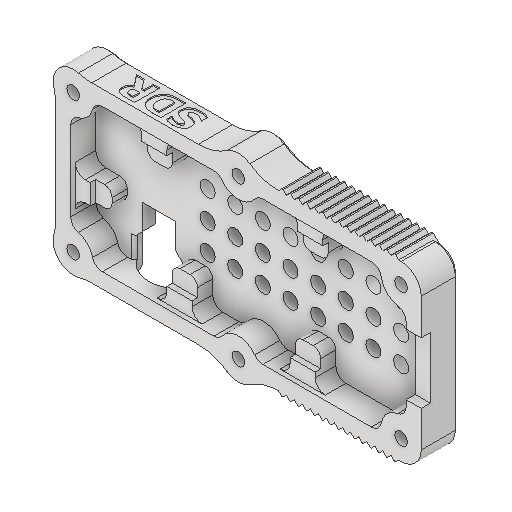
# Autodesk Inventor part: 3DP_PLA_Case_bottom_half
Saved by Autodesk Inventor 2025 (Build 290162010, 162A)
## iProperties
Created: 2018-09-08
Part Number: 3DP_PLA_Case_bottom_half
Material: ABS Plastic
Document SubType Name: Modeling
Designer: Andrzej
Density: 1.06 g/cm^3
Appearance: Smooth - White
Author: Andrzej
Autodesk Inventor part; units mm, degrees
ref_plane "YZ Plane" through (0, 0, 0) normal (1, 0, 0) x (0, 1, 0)
ref_plane "XZ Plane" through (0, 0, 0) normal (0, 1, 0) x (-1, 0, 0)
ref_plane "XY Plane" through (0, 0, 0) normal (0, 0, 1) x (1, 0, 0)
sketch "Sketch1" plane through (0, 0, 0) normal (0, 0, 1) x (1, 0, 0)
  line L0 (-16.557, 11) -> (35.343, 11)
  line L1 (35.343, -11) -> (-16.557, -11)
  line L2 (-20.157, -7.4) -> (-20.157, 7.4)
  line L3 (38.843, 7) -> (46.2445, 7)
  line L4 (46.2445, 7) -> (46.2445, -7)
  line L5 (46.2445, -7) -> (38.843, -7)
  arc A0 (-20.157, -7.4) -> (-16.557, -11) centre (-16.557, -7.4) ccw
  arc A1 (-16.557, 11) -> (-20.157, 7.4) centre (-16.557, 7.4) ccw
  arc A2 (37.843, 8.5) -> (35.343, 11) centre (35.343, 8.5) ccw
  arc A3 (35.343, -11) -> (37.843, -8.5) centre (35.343, -8.5) ccw
  line L6 (37.843, 8.5) -> (37.843, 8)
  line L7 (37.843, -8) -> (37.843, -8.5)
  arc A4 (37.843, 8) -> (38.843, 7) centre (38.843, 8) ccw
  arc A5 (38.843, -7) -> (37.843, -8) centre (38.843, -8) ccw
  circle A6 centre (-17.157, -8) radius 1.05
  circle A7 centre (-15.157, 9.4) radius 1.05
  line L8 (-5.157, -11) -> (-0.157, -11)
  line L9 (-0.157, -11) -> (-0.157, -8)
  line L10 (-0.157, -8) -> (-5.157, -8)
  line L11 (-5.157, -8) -> (-5.157, -11)
  line L12 (19.343, -11) -> (24.343, -11)
  line L13 (24.343, -11) -> (24.343, -8)
  line L14 (24.343, -8) -> (19.343, -8)
  line L15 (19.343, -8) -> (19.343, -11)
  line L16 (-10.157, 11) -> (-5.157, 11)
  line L17 (-5.157, 11) -> (-5.157, 8)
  line L18 (-5.157, 8) -> (-10.157, 8)
  line L19 (-10.157, 8) -> (-10.157, 11)
  line L20 (20.843, 11) -> (25.843, 11)
  line L21 (25.843, 11) -> (25.843, 8)
  line L22 (25.843, 8) -> (20.843, 8)
  line L23 (20.843, 8) -> (20.843, 11)
  line L24 (-10.157, 11) -> (-5.157, 11)
  line L25 (-5.157, 11) -> (-5.157, 11.25)
  line L26 (-5.157, 11.25) -> (-10.157, 11.25)
  line L27 (-10.157, 11.25) -> (-10.157, 11)
  line L28 (20.843, 11) -> (25.843, 11)
  line L29 (25.843, 11) -> (25.843, 11.25)
  line L30 (25.843, 11.25) -> (20.843, 11.25)
  line L31 (20.843, 11.25) -> (20.843, 11)
  line L32 (-5.157, -11) -> (-0.157, -11)
  line L33 (-0.157, -11) -> (-0.157, -11.25)
  line L34 (-0.157, -11.25) -> (-5.157, -11.25)
  line L35 (-5.157, -11.25) -> (-5.157, -11)
  line L36 (19.343, -11) -> (24.343, -11)
  line L37 (24.343, -11) -> (24.343, -11.25)
  line L38 (24.343, -11.25) -> (19.343, -11.25)
  line L39 (19.343, -11.25) -> (19.343, -11)
  line L40 (-5.157, -11.25) -> (-0.157, -11.25)
  line L41 (-0.157, -11.25) -> (-0.157, -14.25)
  line L42 (-0.157, -14.25) -> (-5.157, -14.25)
  line L43 (-5.157, -14.25) -> (-5.157, -11.25)
  line L44 (19.343, -11.25) -> (24.343, -11.25)
  line L45 (24.343, -11.25) -> (24.343, -14.25)
  line L46 (24.343, -14.25) -> (19.343, -14.25)
  line L47 (19.343, -14.25) -> (19.343, -11.25)
  line L48 (-10.157, 11.25) -> (-5.157, 11.25)
  line L49 (-5.157, 11.25) -> (-5.157, 14.25)
  line L50 (-5.157, 14.25) -> (-10.157, 14.25)
  line L51 (-10.157, 14.25) -> (-10.157, 11.25)
  line L52 (20.843, 11.25) -> (25.843, 11.25)
  line L53 (25.843, 11.25) -> (25.843, 14.25)
  line L54 (25.843, 14.25) -> (20.843, 14.25)
  line L55 (20.843, 14.25) -> (20.843, 11.25)
  line L56 (-20.157, -5) -> (-17.157, -5)
  line L57 (-17.157, -5) -> (-17.157, -1)
  line L58 (-17.157, -1) -> (-20.157, -1)
  line L59 (-20.157, -1) -> (-20.157, -5)
  line L60 (-20.157, -5) -> (-20.407, -5)
  line L61 (-20.407, -5) -> (-20.407, -1)
  line L62 (-20.407, -1) -> (-20.157, -1)
  line L63 (-20.157, -1) -> (-20.157, -5)
  line L64 (-20.407, -1) -> (-23.407, -1)
  line L65 (-23.407, -1) -> (-23.407, -5)
  line L66 (-23.407, -5) -> (-20.407, -5)
  line L67 (-20.407, -5) -> (-20.407, -1)
  point P0 (0, 0)
  point P1 (0, 0)
  dimension "d0" = 14
  dimension "d1" = 4
  dimension "d2" = 3.6
  dimension "d3" = 2.5
  dimension "d4" = 1
  dimension "d5" = 2.1
  dimension "d6" = 3
  dimension "d7" = 3
  dimension "d8" = 2.1
  dimension "d9" = 5
  dimension "d10" = 1.6
  dimension "d12" = 5
  dimension "d13" = 3
  dimension "d14" = 5
  dimension "d15" = 3
  dimension "d16" = 5
  dimension "d17" = 3
  dimension "d18" = 5
  dimension "d19" = 3
  dimension "d20" = 15
  dimension "d21" = 10
  dimension "d22" = 5
  dimension "d23" = 0.25
  dimension "d24" = 5
  dimension "d25" = 0.25
  dimension "d27" = 5
  dimension "d28" = 0.25
  dimension "d29" = 5
  dimension "d30" = 0.25
  dimension "d31" = 3
  dimension "d32" = 5
  dimension "d33" = 3
  dimension "d34" = 5
  dimension "d35" = 3
  dimension "d36" = 5
  dimension "d37" = 3
  dimension "d42" = 22
  dimension "d43" = 3
  dimension "d44" = 4
  dimension "d45" = 0.25
  dimension "d46" = 3
  dimension "d47" = 6
  dimension "d69" = 58
  dimension "d70" = 12
  dimension "d71" = 5
  dimension "d72" = 13.5
  dimension "d148" = 11
  constraints: 136 end point, 33 parallel, 20 perpendicular, 17 horizontal, 14 tangent, 12 point on circle, 8 centre point, 7 point on line, 3 equal radius
  measures "d0" distance of L3.end L4.end
  measures "d1" distance between parallel lines of L0 L3
  measures "d2" radius of A0
  measures "d3" radius of A2
  measures "d4" radius of A4
  measures "d5" diameter of A6
  measures "d6" distance from line of L1 A6.centre
  measures "d7" distance from line of L2 A6.centre
  measures "d8" diameter of A7
  measures "d9" distance from line of L2 A7.centre
  measures "d10" distance from line of L0 A7.centre
  measures "d12" distance of L10.end L9.end
  measures "d13" distance of L9.end L8.end
  measures "d14" distance of L14.end L13.end
  measures "d15" distance of L13.end L12.end
  measures "d16" distance of L17.end L18.end
  measures "d17" distance of L16.end L17.end
  measures "d18" distance of L21.end L22.end
  measures "d19" distance of L20.end L21.end
  measures "d20" distance between parallel lines of L2 L11
  measures "d21" distance between parallel lines of L2 L19
  measures "d22" distance of L26.end L25.end
  measures "d23" distance of L25.end L24.end
  measures "d24" distance of L30.end L29.end
  measures "d25" distance of L29.end L28.end
  measures "d27" distance of L33.end L34.end
  measures "d28" distance of L32.end L33.end
  measures "d29" distance of L37.end L38.end
  measures "d30" distance of L36.end L37.end
  measures "d31" distance of L40.end L41.end
  measures "d32" distance of L45.end L46.end
  measures "d33" distance of L44.end L45.end
  measures "d34" distance of L50.end L49.end
  measures "d35" distance of L49.end L48.end
  measures "d36" distance of L54.end L53.end
  measures "d37" distance of L53.end L52.end
  measures "d42" distance between parallel lines of L1 L0
  measures "d43" distance of L58.end L57.end
  measures "d44" distance of L57.end L56.end
  measures "d45" distance of L61.end L62.end
  measures "d46" distance of L66.end L65.end
  measures "d47" distance between parallel lines of L1 L56
  measures "d69" distance between parallel lines of L2 L6
  measures "d70" distance between parallel lines of L6 L21
  measures "d71" distance of L41.end L42.end
  measures "d72" distance between parallel lines of L7 L13
  measures "d148" distance from line of point (0, 0) L0
extrude "Extrusion1" add sketch "Sketch1" against normal blind 3 contours L27 L26 L25 L0 | L0 L17 L18 L19 | L51 L50 L49 L26 | L58 L57 L56 L2 | L2 L60 L61 L62 | L31 L30 L29 L0 | L0 L21 L22 L23 | L61 L66 L65 L64 | L55 L54 L53 L30 | L11 L10 L9 L1 | L1 L33 L34 L35 | L34 L41 L42 L43 | L15 L14 L13 L1 | L1 L37 L38 L39 | L38 L45 L46 L47
extrude "Extrusion2" add sketch "Sketch1" along normal blind 1.1 contours L51 L50 L49 L26 | L61 L66 L65 L64 | L55 L54 L53 L30 | L34 L41 L42 L43 | L38 L45 L46 L47
sketch "Sketch2" plane through (0, 0, -3) normal (0, 0, -1) x (-1, 0, 0)
  line L0 (17.157, -5) -> (23.407, -5) projected
  line L1 (23.407, -5) -> (23.407, -1) projected
  line L2 (23.407, -1) -> (17.157, -1) projected
  line L3 (17.157, -1) -> (17.157, -5) projected
  line L4 (5.157, -14.25) -> (5.157, -8) projected
  line L5 (5.157, -8) -> (0.157, -8) projected
  line L6 (0.157, -8) -> (0.157, -14.25) projected
  line L7 (0.157, -14.25) -> (5.157, -14.25) projected
  line L8 (-19.343, -14.25) -> (-19.343, -8) projected
  line L9 (-19.343, -8) -> (-24.343, -8) projected
  line L10 (-24.343, -8) -> (-24.343, -14.25) projected
  line L11 (-24.343, -14.25) -> (-19.343, -14.25) projected
  line L12 (-20.843, 8) -> (-20.843, 14.25) projected
  line L13 (-20.843, 14.25) -> (-25.843, 14.25) projected
  line L14 (-25.843, 14.25) -> (-25.843, 8) projected
  line L15 (-25.843, 8) -> (-20.843, 8) projected
  line L16 (10.157, 8) -> (10.157, 14.25) projected
  line L17 (10.157, 14.25) -> (5.157, 14.25) projected
  line L18 (5.157, 14.25) -> (5.157, 8) projected
  line L19 (5.157, 8) -> (10.157, 8) projected
  line L20 (23.407, 14.25) -> (-46.343, 14.25)
  line L21 (-46.343, 14.25) -> (-46.343, -14.25)
  line L22 (-46.343, -14.25) -> (23.407, -14.25)
  line L23 (23.407, -14.25) -> (23.407, 14.25)
  line L24 (23.407, -5) -> (23.407, -1) projected
  line L25 (0.157, -14.25) -> (5.157, -14.25) projected
  line L26 (-46.343, -14.25) -> (-46.343, -17.25)
  line L27 (-46.343, -17.25) -> (26.407, -17.25)
  line L28 (26.407, -17.25) -> (26.407, 17.25)
  line L29 (26.407, 17.25) -> (-46.343, 17.25)
  line L30 (-46.343, 17.25) -> (-46.343, 14.25)
  dimension "d49" = 28.5
  dimension "d50" = 47.75
  dimension "d51" = 28.5
  dimension "d52" = 69.75
  dimension "d53" = 3
  dimension "d54" = 3
  dimension "d55" = 3
  constraints: 18 end point, 4 perpendicular, 3 collinear, 2 parallel, 1 horizontal, 1 point on line, 1 vertical
  measures "d49" distance between parallel lines of L17 L7
  measures "d50" distance between parallel lines of L10 L1
  measures "d51" distance of L20.end L21.end
  measures "d52" distance of L21.end L22.end
  measures "d53" distance between parallel lines of L27 L22
  measures "d54" distance between parallel lines of L20 L29
  measures "d55" distance between parallel lines of L28 L23
extrude "Extrusion3" add sketch "Sketch2" along normal blind 2.5
sketch "Sketch3" plane through (0, 0, -3) normal (0, 0, 1) x (1, 0, 0)
  line L0 (46.343, 17.25) -> (46.343, -17.25) projected
  line L1 (-26.407, 17.25) -> (46.343, 17.25) projected
  line L2 (-26.407, -17.25) -> (-26.407, 17.25) projected
  line L3 (46.343, -17.25) -> (-26.407, -17.25) projected
  line L4 (24.343, -14.25) -> (19.343, -14.25) projected
  line L5 (19.343, -14.25) -> (19.343, -8) projected
  line L6 (19.343, -8) -> (24.343, -8) projected
  line L7 (24.343, -8) -> (24.343, -14.25) projected
  line L8 (-10.157, 14.25) -> (-5.157, 14.25) projected
  line L9 (-5.157, 14.25) -> (-5.157, 8) projected
  line L10 (-5.157, 8) -> (-10.157, 8) projected
  line L11 (-10.157, 8) -> (-10.157, 14.25) projected
  line L12 (-23.407, -5) -> (-23.407, -1) projected
  line L13 (-23.407, -1) -> (-17.157, -1) projected
  line L14 (-17.157, -1) -> (-17.157, -5) projected
  line L15 (-17.157, -5) -> (-23.407, -5) projected
  line L16 (20.843, 14.25) -> (25.843, 14.25) projected
  line L17 (25.843, 14.25) -> (25.843, 8) projected
  line L18 (25.843, 8) -> (20.843, 8) projected
  line L19 (20.843, 8) -> (20.843, 14.25) projected
  line L20 (-0.157, -14.25) -> (-5.157, -14.25) projected
  line L21 (-5.157, -14.25) -> (-5.157, -8) projected
  line L22 (-5.157, -8) -> (-0.157, -8) projected
  line L23 (-0.157, -8) -> (-0.157, -14.25) projected
  line L24 (43.343, 14.25) -> (43.343, -14.25)
  line L25 (43.343, -14.25) -> (-23.407, -14.25)
  line L26 (-23.407, -14.25) -> (-23.407, 14.25)
  line L27 (-23.407, 14.25) -> (43.343, 14.25)
  dimension "d58" = 3
  constraints: 8 end point, 3 other
  measures "d58" distance between parallel lines of L1 L27
extrude "Extrusion4" add sketch "Sketch3" along normal blind 5
fillet "Fillet1" radius 6 4 edges at (-23.407, 14.25, -0.5) (-26.407, 17.25, -1.75) (-23.407, -14.25, -0.5) (-26.407, -17.25, -1.75)
fillet "Fillet1" radius 4 4 edges at (43.343, 14.25, -0.5) (46.343, 17.25, -1.75) (46.343, -17.25, -1.75) (43.343, -14.25, -0.5)
sketch "Sketch5" plane through (0, 0, 2) normal (0, 0, 1) x (1, 0, 0)
  line L0 (39.343, -14.25) -> (-17.407, -14.25) projected
  arc A0 (-23.407, -8.25) -> (-17.407, -14.25) centre (-17.407, -8.25) ccw projected
  line L1 (-23.407, -8.25) -> (-23.407, 8.25) projected
  arc A1 (-17.407, 14.25) -> (-23.407, 8.25) centre (-17.407, 8.25) ccw projected
  line L2 (-17.407, 14.25) -> (39.343, 14.25) projected
  arc A2 (43.343, 10.25) -> (39.343, 14.25) centre (39.343, 10.25) ccw projected
  line L3 (43.343, 10.25) -> (43.343, -10.25) projected
  arc A3 (39.343, -14.25) -> (43.343, -10.25) centre (39.343, -10.25) ccw projected
  arc A4 (42.343, -17.25) -> (46.343, -13.25) centre (42.343, -13.25) ccw projected
  line L4 (46.343, -13.25) -> (46.343, 13.25) projected
  arc A5 (46.343, 13.25) -> (42.343, 17.25) centre (42.343, 13.25) ccw projected
  line L5 (42.343, 17.25) -> (-20.407, 17.25) projected
  arc A6 (-20.407, 17.25) -> (-26.407, 11.25) centre (-20.407, 11.25) ccw projected
  line L6 (-26.407, 11.25) -> (-26.407, -11.25) projected
  arc A7 (-26.407, -11.25) -> (-20.407, -17.25) centre (-20.407, -11.25) ccw projected
  line L7 (-20.407, -17.25) -> (42.343, -17.25) projected
  circle A8 centre (42.343, -13.25) radius 4
  circle A9 centre (9.968, -15.75) radius 4
  circle A10 centre (-22.907, -13.75) radius 4
  circle A11 centre (42.343, 13.25) radius 4
  circle A12 centre (9.968, 15.75) radius 4
  circle A13 centre (-22.907, 13.75) radius 4
  point P0 (0, 0)
  dimension "d73" = 8
  dimension "d74" = 8
  dimension "d75" = 8
  dimension "d76" = 36.375
  dimension "d77" = 72.75
  dimension "d78" = 1.5
  dimension "d79" = 8
  dimension "d80" = 8
  dimension "d81" = 8
  dimension "d82" = 3.5
  dimension "d83" = 3.5
  dimension "d84" = 3.5
  dimension "d85" = 1.5
  constraints: 6 centre point, 2 coincident, 2 vertical alignment
  measures "d73" diameter of A8
  measures "d74" diameter of A9
  measures "d75" diameter of A10
  measures "d76" distance from line of L4 A9.centre
  measures "d77" distance between parallel lines of L4 L6
  measures "d78" distance from line of L7 A9.centre
  measures "d79" diameter of A11
  measures "d80" diameter of A12
  measures "d81" diameter of A13
  measures "d82" distance from line of A10.centre L7
  measures "d83" distance from line of A10.centre L6
  measures "d84" distance from line of L5 A13.centre
  measures "d85" distance from line of L5 A12.centre
extrude "Extrusion5" add sketch "Sketch5" against normal up to surface (7.5 mm away) contours A3 L3 A8 A4 L0 | L0 A8 L3 A3 | A9 L7 L0 | L0 A9 | A11 L2 A2 L3 | L3 A2 L2 A11 A5 | A9 L7 | A10 A7 A0 | A0 A10 | A12 L2 | L2 A12 L5 | A10 A7 | L5 A12 | A13 A1 | A1 A13 A6 | A6 A13
hole "Hole1" at (-22.907, -13.75, 2) at (9.968, -15.75, 2) at (42.343, -13.25, 2) at (9.968, 15.75, 2) at (42.343, 13.25, 2) at (-22.907, 13.75, 2) direction (0, 0, -1) diameter 2.5 end through all both
sketch "Sketch6" plane through (46.343, -13.25, -5.5) normal (1, 0, 0) x (0, 0, -1)
  line L0 (0, 0) -> (-7.5, 0) projected
  line L1 (0, 26.5) -> (0, 0) projected
  line L2 (-7.5, 26.5) -> (0, 26.5) projected
  line L3 (-7.5, 0) -> (-7.5, 26.5) projected
  line L4 (-7.5, 22.627) -> (-7.5, 3.873) projected
  line L5 (-7.5, 7.175) -> (-5.7, 7.175)
  line L6 (-5.7, 7.175) -> (-5.7, 19.325)
  line L7 (-5.7, 19.325) -> (-7.5, 19.325)
  line L8 (-7.5, 7.175) -> (-7.5, 19.325)
  point P0 (-5.5, 13.25)
  dimension "d95" = 1.8
  dimension "d96" = 12.15
  dimension "d97" = 26.5
  dimension "d98" = 7.175
  constraints: 8 end point, 2 perpendicular, 2 point on line, 1 collinear, 1 horizontal
  measures "d95" distance of L5.start L5.end
  measures "d96" distance of L5.end L6.end
  measures "d97" distance between parallel lines of L2 L0
  measures "d98" distance between parallel lines of L0 L5
extrude "Extrusion6" cut sketch "Sketch6" against normal blind 6 contours L3 L7 L6 L5
fillet "Fillet2" radius 2 10 edges at (-10.157, 14.25, -0.95) (-5.157, 14.25, -0.95) (20.843, 14.25, -0.95) (25.843, 14.25, -0.95) (19.343, -14.25, -0.95) (24.343, -14.25, -0.95) (-0.157, -14.25, -0.95) (-5.157, -14.25, -0.95) (-23.407, -1, -0.95) (-23.407, -5, -0.95)
fillet "Fillet2" radius 1.5 10 edges at (-10.157, 8, -1.5) (-5.157, 8, -1.5) (20.843, 8, -1.5) (25.843, 8, -1.5) (-17.157, -5, -1.5) (-17.157, -1, -1.5) (-5.157, -8, -1.5) (-0.157, -8, -1.5) (19.343, -8, -1.5) (24.343, -8, -1.5)
sketch "Sketch7" plane through (-20.407, -17.25, -5.5) normal (0, -1, 0) x (1, 0, 0)
  circle A0 centre (9.5728, -1.45) radius 6
  line L0 (26.6669, 0) -> (0, 0) projected
  line L1 (-5.9772, 0) -> (-5.9772, 7.5) projected
  point P0 (20.407, 5.5)
  dimension "d103" = 12
  dimension "d104" = 1.45
  dimension "d105" = 15.55
  constraints: 1 centre point
  measures "d103" diameter of A0
  measures "d104" distance from line of L0 A0.centre
  measures "d105" distance from line of L1 A0.centre
extrude "Extrusion7" cut sketch "Sketch7" against normal blind 7.45
sketch "Sketch8" plane through (0, 0, -5.5) normal (0, 0, -1) x (-1, 0, 0)
  line L0 (5.012, -17.25) -> (5.012, -9.8) projected
  line L1 (5.012, -9.8) -> (16.6563, -9.8) projected
  line L2 (16.6563, -9.8) -> (16.6563, -17.25) projected
  line L3 (16.6563, -17.25) -> (20.407, -17.25) projected
  arc A0 (20.407, -17.25) -> (20.9298, -17.2272) centre (20.407, -11.25) ccw projected
  arc A1 (20.9298, -17.2272) -> (26.3842, -11.7728) centre (22.907, -13.75) ccw projected
  arc A2 (26.3842, -11.7728) -> (26.407, -11.25) centre (20.407, -11.25) ccw projected
  line L4 (26.407, -11.25) -> (26.407, 11.25) projected
  arc A3 (26.407, 11.25) -> (26.3842, 11.7728) centre (20.407, 11.25) ccw projected
  arc A4 (26.3842, 11.7728) -> (20.9298, 17.2272) centre (22.907, 13.75) ccw projected
  arc A5 (20.9298, 17.2272) -> (20.407, 17.25) centre (20.407, 11.25) ccw projected
  line L5 (20.407, 17.25) -> (-6.2599, 17.25) projected
  arc A6 (-6.2599, 17.25) -> (-13.6761, 17.25) centre (-9.968, 15.75) ccw projected
  line L6 (-13.6761, 17.25) -> (-42.343, 17.25) projected
  arc A7 (-42.343, 17.25) -> (-46.343, 13.25) centre (-42.343, 13.25) ccw projected
  line L7 (-46.343, 13.25) -> (-46.343, -13.25) projected
  arc A8 (-46.343, -13.25) -> (-42.343, -17.25) centre (-42.343, -13.25) ccw projected
  line L8 (-42.343, -17.25) -> (-13.6761, -17.25) projected
  arc A9 (-13.6761, -17.25) -> (-6.2599, -17.25) centre (-9.968, -15.75) ccw projected
  line L9 (-6.2599, -17.25) -> (5.012, -17.25) projected
  circle A10 centre (22.907, 13.75) radius 1.25 projected
  circle A11 centre (-9.968, 15.75) radius 1.25 projected
  circle A12 centre (-9.968, -15.75) radius 1.25 projected
  circle A13 centre (22.907, -13.75) radius 1.25 projected
  circle A14 centre (-42.343, -13.25) radius 1.25 projected
  circle A15 centre (-42.343, 13.25) radius 1.25 projected
  line L10 (14.0842, -9.8) -> (7.5842, -9.8)
  line L11 (7.5842, -9.8) -> (7.5842, -3.3)
  line L12 (7.5842, -3.3) -> (14.0842, -3.3)
  line L13 (14.0842, -3.3) -> (14.0842, -9.8)
  point P0 (0, 0)
  dimension "d108" = 6.5
  dimension "d109" = 6.5
  dimension "d110" = 11.6443
  dimension "d111" = 2.5722
  constraints: 8 end point, 2 parallel, 1 horizontal, 1 perpendicular, 1 point on line
  measures "d108" distance of L11.end L12.end
  measures "d109" distance of L10.end L11.end
  measures "d110" distance between parallel lines of L0 L2
  measures "d111" distance between parallel lines of L2 L13
extrude "Extrusion8" cut sketch "Sketch8" against normal blind 8 contours L11 L12 L13 L1
fillet "Fillet3" radius 0.5 2 edges at (-15.3505, -12.025, -3) (-6.3178, -11.9327, -3)
chamfer "Chamfer1" distance 1.5 angle 45 2 edges at (-7.5842, -9.8, -4.25) (-14.0842, -9.8, -4.25)
fillet "Fillet4" radius 10 8 edges at (-26.3842, -11.7728, -1.75) (-26.3842, 11.7728, -1.75) (-20.9298, -17.2272, -1.75) (6.2599, -17.25, -1.75) (13.6761, -17.25, -1.75) (13.6761, 17.25, -1.75) (6.2599, 17.25, -1.75) (-20.9298, 17.2272, -1.75)
sketch "Sketch9" plane through (0, 0, -3) normal (0, 0, 1) x (1, 0, 0)
  line L0 (-14.0842, -8.3) -> (-15.5842, -9.8) projected
  line L1 (-14.0842, -8.3) -> (-14.0842, -3.3) projected
  line L2 (-14.0842, -3.3) -> (-7.5842, -3.3) projected
  line L3 (-7.5842, -3.3) -> (-7.5842, -8.3) projected
  line L4 (-6.0842, -9.8) -> (-7.5842, -8.3) projected
  line L5 (-6.0842, -9.8) -> (-5.3253, -9.8) projected
  line L6 (-5.3253, -13.0531) -> (-5.3253, -9.8) projected
  arc A0 (-5.3253, -13.0531) -> (-5.157, -12.25) centre (-7.157, -12.25) ccw projected
  line L7 (-5.157, -12.25) -> (-5.157, -9.5) projected
  arc A1 (-3.657, -8) -> (-5.157, -9.5) centre (-3.657, -9.5) ccw projected
  line L8 (-3.657, -8) -> (-1.657, -8) projected
  arc A2 (-0.157, -9.5) -> (-1.657, -8) centre (-1.657, -9.5) ccw projected
  line L9 (-0.157, -9.5) -> (-0.157, -12.25) projected
  arc A3 (-0.157, -12.25) -> (1.843, -14.25) centre (1.843, -12.25) ccw projected
  line L10 (1.843, -14.25) -> (6.2599, -14.25) projected
  arc A4 (13.6761, -14.25) -> (6.2599, -14.25) centre (9.968, -15.75) ccw projected
  line L11 (13.6761, -14.25) -> (17.343, -14.25) projected
  arc A5 (17.343, -14.25) -> (19.343, -12.25) centre (17.343, -12.25) ccw projected
  line L12 (19.343, -12.25) -> (19.343, -9.5) projected
  arc A6 (20.843, -8) -> (19.343, -9.5) centre (20.843, -9.5) ccw projected
  line L13 (20.843, -8) -> (22.843, -8) projected
  arc A7 (24.343, -9.5) -> (22.843, -8) centre (22.843, -9.5) ccw projected
  line L14 (24.343, -9.5) -> (24.343, -12.25) projected
  arc A8 (24.343, -12.25) -> (26.343, -14.25) centre (26.343, -12.25) ccw projected
  line L15 (26.343, -14.25) -> (38.47, -14.25) projected
  arc A9 (43.343, -9.377) -> (38.47, -14.25) centre (42.343, -13.25) ccw projected
  line L16 (43.343, -9.377) -> (43.343, 9.377) projected
  arc A10 (38.47, 14.25) -> (43.343, 9.377) centre (42.343, 13.25) ccw projected
  line L17 (38.47, 14.25) -> (27.843, 14.25) projected
  arc A11 (27.843, 14.25) -> (25.843, 12.25) centre (27.843, 12.25) ccw projected
  line L18 (25.843, 12.25) -> (25.843, 9.5) projected
  arc A12 (24.343, 8) -> (25.843, 9.5) centre (24.343, 9.5) ccw projected
  line L19 (24.343, 8) -> (22.343, 8) projected
  arc A13 (20.843, 9.5) -> (22.343, 8) centre (22.343, 9.5) ccw projected
  line L20 (20.843, 9.5) -> (20.843, 12.25) projected
  arc A14 (20.843, 12.25) -> (18.843, 14.25) centre (18.843, 12.25) ccw projected
  line L21 (18.843, 14.25) -> (13.6761, 14.25) projected
  arc A15 (6.2599, 14.25) -> (13.6761, 14.25) centre (9.968, 15.75) ccw projected
  line L22 (6.2599, 14.25) -> (-3.157, 14.25) projected
  arc A16 (-3.157, 14.25) -> (-5.157, 12.25) centre (-3.157, 12.25) ccw projected
  line L23 (-5.157, 12.25) -> (-5.157, 9.5) projected
  arc A17 (-6.657, 8) -> (-5.157, 9.5) centre (-6.657, 9.5) ccw projected
  line L24 (-6.657, 8) -> (-8.657, 8) projected
  arc A18 (-10.157, 9.5) -> (-8.657, 8) centre (-8.657, 9.5) ccw projected
  line L25 (-10.157, 9.5) -> (-10.157, 12.25) projected
  arc A19 (-10.157, 12.25) -> (-12.157, 14.25) centre (-12.157, 12.25) ccw projected
  line L26 (-12.157, 14.25) -> (-17.407, 14.25) projected
  arc A20 (-17.407, 14.25) -> (-18.9187, 14.0564) centre (-17.407, 8.25) ccw projected
  arc A21 (-23.2134, 9.7618) -> (-18.9187, 14.0564) centre (-22.907, 13.75) ccw projected
  arc A22 (-23.2134, 9.7618) -> (-23.407, 8.25) centre (-17.407, 8.25) ccw projected
  line L27 (-23.407, 8.25) -> (-23.407, 1) projected
  arc A23 (-23.407, 1) -> (-21.407, -1) centre (-21.407, 1) ccw projected
  line L28 (-21.407, -1) -> (-18.657, -1) projected
  arc A24 (-17.157, -2.5) -> (-18.657, -1) centre (-18.657, -2.5) ccw projected
  line L29 (-17.157, -2.5) -> (-17.157, -3.5) projected
  arc A25 (-18.657, -5) -> (-17.157, -3.5) centre (-18.657, -3.5) ccw projected
  line L30 (-18.657, -5) -> (-21.407, -5) projected
  arc A26 (-21.407, -5) -> (-23.407, -7) centre (-21.407, -7) ccw projected
  line L31 (-23.407, -7) -> (-23.407, -8.25) projected
  arc A27 (-23.407, -8.25) -> (-23.2134, -9.7618) centre (-17.407, -8.25) ccw projected
  arc A28 (-18.9187, -14.0564) -> (-23.2134, -9.7618) centre (-22.907, -13.75) ccw projected
  arc A29 (-18.9187, -14.0564) -> (-17.407, -14.25) centre (-17.407, -8.25) ccw projected
  line L32 (-17.407, -14.25) -> (-16.343, -14.25) projected
  line L33 (-16.343, -9.8) -> (-16.343, -14.25) projected
  line L34 (-16.343, -9.8) -> (-15.5842, -9.8) projected
  circle A30 centre (37.343, 5.5) radius 1.5
  circle A31 centre (31.843, 5.5) radius 1.5
  circle A32 centre (26.343, 5.5) radius 1.5
  circle A33 centre (20.843, 5.5) radius 1.5
  circle A34 centre (15.343, 5.5) radius 1.5
  circle A35 centre (9.843, 5.5) radius 1.5
  circle A36 centre (4.343, 5.5) radius 1.5
  circle A37 centre (37.343, 0) radius 1.5
  circle A38 centre (31.843, 0) radius 1.5
  circle A39 centre (26.343, 0) radius 1.5
  circle A40 centre (20.843, 0) radius 1.5
  circle A41 centre (15.343, 0) radius 1.5
  circle A42 centre (9.843, 0) radius 1.5
  circle A43 centre (4.343, 0) radius 1.5
  circle A44 centre (37.343, -5.5) radius 1.5
  circle A45 centre (31.843, -5.5) radius 1.5
  circle A46 centre (26.343, -5.5) radius 1.5
  circle A47 centre (20.843, -5.5) radius 1.5
  circle A48 centre (15.343, -5.5) radius 1.5
  circle A49 centre (9.843, -5.5) radius 1.5
  circle A50 centre (4.343, -5.5) radius 1.5
  circle A51 centre (-1.157, 5.5) radius 1.5
  circle A52 centre (-1.157, 0) radius 1.5
  circle A53 centre (-1.157, -5.5) radius 1.5
  point P0 (0, 0)
  dimension "d119" = 3
  dimension "d120" = 6
  dimension "d121" = 8.75
  dimension "d124" = 5.5
  dimension "d127" = 5.5
  constraints: 24 centre point, 1 horizontal, 1 vertical, 46 other
  measures "d119" diameter of A30
  measures "d120" distance from line of L16 A30.centre
  measures "d121" distance from line of L17 A30.centre
  measures "d124" distance of A30.centre A31.centre
  measures "d127" distance of A30.centre A37.centre
extrude "Extrusion9" cut sketch "Sketch9" against normal blind 8 contours A30 | A31 | A32 | A33 | A34 | A35 | A36 | A37 | A38 | A39 | A40 | A41 | A42 | A43 | A44 | A45 | A46 | A47 | A48 | A49 | A50 | A51 | A52 | A53
fillet "Fillet5" radius 2 12 edges at (-18.9187, 14.0564, -0.5) (-23.2134, 9.7618, -0.5) (6.2599, 14.25, -0.5) (13.6761, 14.25, -0.5) (43.343, 9.377, -0.5) (38.47, 14.25, -0.5) (38.47, -14.25, -0.5) (43.343, -9.377, -0.5) (6.2599, -14.25, -0.5) (13.6761, -14.25, -0.5) (-18.9187, -14.0564, -0.5) (-23.2134, -9.7618, -0.5)
sketch "Sketch10" plane through (0, 0, 2) normal (0, 0, 1) x (1, 0, 0)
  arc A0 (-19.034, -12.75) -> (-17.0975, -14.25) centre (-17.0975, -12.25) ccw projected
  arc A1 (-19.034, -12.75) -> (-21.907, -9.877) centre (-22.907, -13.75) ccw projected
  arc A2 (-23.407, -7.9405) -> (-21.907, -9.877) centre (-21.407, -7.9405) ccw projected
  line L0 (-23.407, -7.9405) -> (-23.407, 7.9405) projected
  arc A3 (-21.907, 9.877) -> (-23.407, 7.9405) centre (-21.407, 7.9405) ccw projected
  arc A4 (-21.907, 9.877) -> (-19.034, 12.75) centre (-22.907, 13.75) ccw projected
  arc A5 (-17.0975, 14.25) -> (-19.034, 12.75) centre (-17.0975, 12.25) ccw projected
  line L1 (-17.0975, 14.25) -> (5.0946, 14.25) projected
  arc A6 (6.7191, 13.4167) -> (5.0946, 14.25) centre (5.0946, 12.25) ccw projected
  arc A7 (6.7191, 13.4167) -> (13.2169, 13.4167) centre (9.968, 15.75) ccw projected
  arc A8 (14.8414, 14.25) -> (13.2169, 13.4167) centre (14.8414, 12.25) ccw projected
  line L2 (14.8414, 14.25) -> (36.4269, 14.25) projected
  arc A9 (38.399, 12.5833) -> (36.4269, 14.25) centre (36.4269, 12.25) ccw projected
  arc A10 (38.399, 12.5833) -> (41.6763, 9.3059) centre (42.343, 13.25) ccw projected
  arc A11 (43.343, 7.3339) -> (41.6763, 9.3059) centre (41.343, 7.3339) ccw projected
  line L3 (43.343, 7.3339) -> (43.343, 6.075) projected
  line L4 (43.343, 6.075) -> (46.343, 6.075) projected
  line L5 (46.343, 6.075) -> (46.343, 13.25) projected
  arc A12 (46.343, 13.25) -> (42.343, 17.25) centre (42.343, 13.25) ccw projected
  line L6 (42.343, 17.25) -> (17.9524, 17.25) projected
  arc A13 (12.2493, 19.0357) -> (17.9524, 17.25) centre (17.9524, 27.25) ccw projected
  arc A14 (12.2493, 19.0357) -> (7.6868, 19.0357) centre (9.968, 15.75) ccw projected
  arc A15 (1.9837, 17.25) -> (7.6868, 19.0357) centre (1.9837, 27.25) ccw projected
  line L7 (1.9837, 17.25) -> (-19.1989, 17.25) projected
  arc A16 (-21.8475, 17.6071) -> (-19.1989, 17.25) centre (-19.1989, 27.25) ccw projected
  arc A17 (-21.8475, 17.6071) -> (-26.7641, 12.6905) centre (-22.907, 13.75) ccw projected
  arc A18 (-26.407, 10.0419) -> (-26.7641, 12.6905) centre (-36.407, 10.0419) ccw projected
  line L8 (-26.407, 10.0419) -> (-26.407, -10.0419) projected
  arc A19 (-26.7641, -12.6905) -> (-26.407, -10.0419) centre (-36.407, -10.0419) ccw projected
  arc A20 (-26.7641, -12.6905) -> (-21.8475, -17.6071) centre (-22.907, -13.75) ccw projected
  arc A21 (-19.1989, -17.25) -> (-21.8475, -17.6071) centre (-19.1989, -27.25) ccw projected
  line L9 (-19.1989, -17.25) -> (1.9837, -17.25) projected
  arc A22 (7.6868, -19.0357) -> (1.9837, -17.25) centre (1.9837, -27.25) ccw projected
  arc A23 (7.6868, -19.0357) -> (12.2493, -19.0357) centre (9.968, -15.75) ccw projected
  arc A24 (17.9524, -17.25) -> (12.2493, -19.0357) centre (17.9524, -27.25) ccw projected
  line L10 (17.9524, -17.25) -> (42.343, -17.25) projected
  arc A25 (42.343, -17.25) -> (46.343, -13.25) centre (42.343, -13.25) ccw projected
  line L11 (46.343, -13.25) -> (46.343, -6.075) projected
  line L12 (46.343, -6.075) -> (43.343, -6.075) projected
  line L13 (43.343, -6.075) -> (43.343, -7.3339) projected
  arc A26 (41.6763, -9.3059) -> (43.343, -7.3339) centre (41.343, -7.3339) ccw projected
  arc A27 (41.6763, -9.3059) -> (38.399, -12.5833) centre (42.343, -13.25) ccw projected
  arc A28 (36.4269, -14.25) -> (38.399, -12.5833) centre (36.4269, -12.25) ccw projected
  line L14 (36.4269, -14.25) -> (14.8414, -14.25) projected
  arc A29 (13.2169, -13.4167) -> (14.8414, -14.25) centre (14.8414, -12.25) ccw projected
  arc A30 (13.2169, -13.4167) -> (6.7191, -13.4167) centre (9.968, -15.75) ccw projected
  arc A31 (5.0946, -14.25) -> (6.7191, -13.4167) centre (5.0946, -12.25) ccw projected
  line L15 (5.0946, -14.25) -> (-17.0975, -14.25) projected
  circle A32 centre (42.343, 13.25) radius 1.25 projected
  circle A33 centre (42.343, -13.25) radius 1.25 projected
  circle A34 centre (-22.907, -13.75) radius 1.25 projected
  circle A35 centre (9.968, -15.75) radius 1.25 projected
  circle A36 centre (9.968, 15.75) radius 1.25 projected
  circle A37 centre (-22.907, 13.75) radius 1.25 projected
  line L16 (17.9524, -17.25) -> (42.343, -17.25) projected
  line L17 (17.9524, -17.25) -> (18.7024, -18)
  line L18 (17.9524, -17.25) -> (19.3124, -17.25) construction
  line L19 (19.4524, -17.25) -> (18.7024, -18)
  line L20 (19.4524, -17.25) -> (21.5024, -17.25) construction
  point P0 (0, 0)
  dimension "d134" = 45
  dimension "d136" = 135
  dimension "d137" = 1.5
  constraints: 8 end point, 2 horizontal, 1 point on line
  measures "d134" angle of L17 L18
  measures "d136" angle of L19 L20
  measures "d137" distance of L10.start L19.start
extrude "Extrusion10" add sketch "Sketch10" against normal up to surface (7.5 mm away) contours L19 L17 L10
fillet "Fillet7" radius 0.2 1 edges at (18.7024, -18, -1.75)
pattern_linear "Rectangular Pattern2" count 15 spacing 1.6 along (1, 0, 0) of "Extrusion10", "Fillet7"
chamfer "Chamfer2" distance 0.5 angle 45 1 edges at (-10.8342, -17.25, -0.95)
mirror "Mirror1" about plane through (0, 0, 0) normal (0, 1, 0) of "Extrusion10", "Fillet7", "Rectangular Pattern2"
chamfer "Chamfer3" distance 0.7 angle 45 21 edges at (-26.407, 0, -5.5) (-26.4967, 11.3782, -5.5) (-25.7354, 16.5784, -5.5) (-20.5352, 17.3397, -5.5) (-8.6076, 17.25, -5.5) (4.9717, 17.7069, -5.5) (9.968, 19.75, -5.5) (14.9643, 17.7069, -5.5) (-26.4967, -11.3782, -5.5) (-25.7354, -16.5784, -5.5) (-20.5352, -17.3397, -5.5) (-18.1846, -17.25, -5.5) (-1.2572, -17.25, -5.5) (4.9717, -17.7069, -5.5) (9.968, -19.75, -5.5) (14.9643, -17.7069, -5.5) (45.1714, 16.0784, -5.5) (42.0977, 17.25, -5.5) (46.343, 0, -5.5) (45.1714, -16.0784, -5.5) (42.0977, -17.25, -5.5)
sketch "Sketch11" plane through (-19.1989, 17.25, 2) normal (0, 1, 0) x (1, 0, 0)
  line L0 (0, 6.8) -> (21.1825, 6.8) projected
  line L1 (0, 0) -> (0, 6.8) projected
  line L2 (21.1825, 0) -> (0, 0) projected
  line L3 (21.1825, 6.8) -> (21.1825, 0) projected
  line L4 (17.7206, 0.769) -> (-4.7017, 0.769) construction
  line L5 (-4.7017, 0.769) -> (-4.7017, 9.6455) construction
  line L6 (-4.7017, 9.6455) -> (17.7206, 9.6455) construction
  line L7 (17.7206, 9.6455) -> (17.7206, 0.769) construction
  spline S0 degree 2 poles (15.6582, 5.9473) (16.2335, 5.9473) (17.1006, 5.7245) (17.4734, 5.5624) knots 0 0 0 1 2 2 2
  line L8 (17.4734, 5.5624) -> (17.4734, 4.3712)
  line L9 (17.4734, 4.3712) -> (17.3599, 4.3712)
  spline S1 degree 2 poles (17.3599, 4.3712) (16.9831, 4.6913) (16.0796, 5.0357) (15.6541, 5.0357) knots 0 0 0 1 2 2 2
  spline S2 degree 2 poles (15.6541, 5.0357) (15.5447, 5.0357) (15.1922, 4.987) (15.0869, 4.9384) knots 0 0 0 1 2 2 2
  spline S3 degree 2 poles (15.0869, 4.9384) (14.9572, 4.8817) (14.7749, 4.675) (14.7749, 4.5089) knots 0 0 0 1 2 2 2
  spline S4 degree 2 poles (14.7749, 4.5089) (14.7749, 4.3185) (15.0706, 4.0835) (15.2732, 4.0308) knots 0 0 0 1 2 2 2
  spline S5 degree 2 poles (15.2732, 4.0308) (15.5285, 3.9619) (16.1079, 3.8444) (16.3632, 3.7553) knots 0 0 0 1 2 2 2
  spline S6 degree 2 poles (16.3632, 3.7553) (16.9426, 3.5527) (17.445, 2.8598) (17.445, 2.3412) knots 0 0 0 1 2 2 2
  spline S7 degree 2 poles (17.445, 2.3412) (17.445, 1.6402) (16.2578, 0.769) (15.3664, 0.769) knots 0 0 0 1 2 2 2
  spline S8 degree 2 poles (15.3664, 0.769) (14.9207, 0.769) (14.0374, 0.9514) (13.689, 1.1054) knots 0 0 0 1 2 2 2
  line L10 (13.689, 1.1054) -> (13.689, 2.248)
  line L11 (13.689, 2.248) -> (13.7984, 2.248)
  spline S9 degree 2 poles (13.7984, 2.248) (14.0779, 2.0089) (14.8802, 1.6807) (15.3016, 1.6807) knots 0 0 0 1 2 2 2
  spline S10 degree 2 poles (15.3016, 1.6807) (15.4677, 1.6807) (15.727, 1.7293) (15.8729, 1.7942) knots 0 0 0 1 2 2 2
  spline S11 degree 2 poles (15.8729, 1.7942) (15.9904, 1.8468) (16.1606, 2.0575) (16.1606, 2.1872) knots 0 0 0 1 2 2 2
  spline S12 degree 2 poles (16.1606, 2.1872) (16.1606, 2.3817) (15.8891, 2.6045) (15.5001, 2.6937) knots 0 0 0 1 2 2 2
  spline S13 degree 2 poles (15.5001, 2.6937) (15.2489, 2.7504) (14.783, 2.8598) (14.5155, 2.953) knots 0 0 0 1 2 2 2
  spline S14 degree 2 poles (14.5155, 2.953) (13.9969, 3.1434) (13.4904, 3.7755) (13.4904, 4.2942) knots 0 0 0 1 2 2 2
  spline S15 degree 2 poles (13.4904, 4.2942) (13.4904, 5.0397) (14.6614, 5.9473) (15.6582, 5.9473) knots 0 0 0 1 2 2 2
  spline S16 degree 2 poles (8.3851, 3.3622) (8.3851, 4.0632) (8.9969, 5.1653) (9.4629, 5.4611) knots 0 0 0 1 2 2 2
  spline S17 degree 2 poles (9.4629, 5.4611) (9.8518, 5.7123) (10.7676, 5.8582) (11.2822, 5.8582) knots 0 0 0 1 2 2 2
  line L12 (11.2822, 5.8582) -> (12.8462, 5.8582)
  line L13 (12.8462, 5.8582) -> (12.8462, 0.8582)
  line L14 (12.8462, 0.8582) -> (11.2984, 0.8582)
  spline S18 degree 2 poles (11.2984, 0.8582) (10.7716, 0.8582) (9.8518, 0.9919) (9.4467, 1.2512) knots 0 0 0 1 2 2 2
  spline S19 degree 2 poles (9.4467, 1.2512) (8.9564, 1.5673) (8.3851, 2.637) (8.3851, 3.3622) knots 0 0 0 1 2 2 2
  spline S20 degree 2 poles (9.6736, 3.3541) (9.6736, 2.8598) (10.0139, 2.1548) (10.3624, 1.9562) knots 0 0 0 1 2 2 2
  spline S21 degree 2 poles (10.3624, 1.9562) (10.6176, 1.8185) (11.1768, 1.7901) (11.5658, 1.7901) knots 0 0 0 1 2 2 2
  line L15 (11.5658, 1.7901) -> (11.5901, 1.7901)
  line L16 (11.5901, 1.7901) -> (11.5901, 4.9222)
  line L17 (11.5901, 4.9222) -> (11.5658, 4.9222)
  spline S22 degree 2 poles (11.5658, 4.9222) (11.1444, 4.9222) (10.565, 4.8938) (10.3016, 4.7277) knots 0 0 0 1 2 2 2
  spline S23 degree 2 poles (10.3016, 4.7277) (9.9937, 4.5332) (9.6736, 3.8485) (9.6736, 3.3541) knots 0 0 0 1 2 2 2
  line L18 (3.0204, 5.8582) -> (4.548, 5.8582)
  line L19 (4.548, 5.8582) -> (5.9377, 4.0227)
  line L20 (5.9377, 4.0227) -> (6.3916, 4.0227)
  line L21 (6.3916, 4.0227) -> (6.3916, 5.8582)
  line L22 (6.3916, 5.8582) -> (7.6395, 5.8582)
  line L23 (7.6395, 5.8582) -> (7.6395, 0.8582)
  line L24 (7.6395, 0.8582) -> (5.6298, 0.8582)
  spline S24 degree 2 poles (5.6298, 0.8582) (5.2125, 0.8582) (4.5966, 0.9635) (4.3332, 1.1256) knots 0 0 0 1 2 2 2
  spline S25 degree 2 poles (4.3332, 1.1256) (4.0658, 1.2958) (3.7497, 1.8266) (3.7497, 2.2318) knots 0 0 0 1 2 2 2
  spline S26 degree 2 poles (3.7497, 2.2318) (3.7497, 2.8031) (4.2684, 3.5203) (4.7019, 3.731) knots 0 0 0 1 2 2 2
  line L25 (4.7019, 3.731) -> (3.0204, 5.8582)
  spline S27 degree 2 poles (5.0382, 2.3898) (5.0382, 2.1994) (5.1841, 1.9279) (5.3502, 1.8549) knots 0 0 0 1 2 2 2
  spline S28 degree 2 poles (5.3502, 1.8549) (5.4677, 1.8063) (5.7554, 1.778) (5.9702, 1.778) knots 0 0 0 1 2 2 2
  line L26 (5.9702, 1.778) -> (6.3916, 1.778)
  line L27 (6.3916, 1.778) -> (6.3916, 3.1232)
  line L28 (6.3916, 3.1232) -> (6.0309, 3.1232)
  spline S29 degree 2 poles (6.0309, 3.1232) (5.7716, 3.1232) (5.4029, 3.0584) (5.2773, 2.9571) knots 0 0 0 1 2 2 2
  spline S30 degree 2 poles (5.2773, 2.9571) (5.1557, 2.8598) (5.0382, 2.6005) (5.0382, 2.3898) knots 0 0 0 1 2 2 2
  point P0 (19.1989, 2)
  constraints: 2 other
extrude "Extrusion11" cut sketch "Sketch11" against normal blind 0.25 contours S0 L8 L9 S1 S2 S3 S4 S5 S6 S7 S8 L10 L11 S9 S10 S11 S12 S13 S14 S15 | S16 S17 L12 L13 L14 S18 S19 | L18 L19 L20 L21 L22 L23 L24 S24 S25 S26 L25
equation "\"d1\" = -0.5 * d0 + 0.5 * d11"
equation "\"d25\" = d23"
equation "\"d28\" = d23"
equation "\"d30\" = d23"
equation "\"d31\" = d35"
equation "\"d33\" = d35"
equation "\"d37\" = d35"
equation "\"d71\" = d27"
equation "\"d51\" = d49"
equation "\"d54\" = d53"
equation "\"d76\" = 0.5 * d77"
equation "\"d83\" = d82"
equation "\"d84\" = d82"
equation "\"d85\" = d78"
equation "\"d98\" = -0.5 * d96 + 0.5 * d97"
equation "\"d11\" = 22"
body "Solid1"
